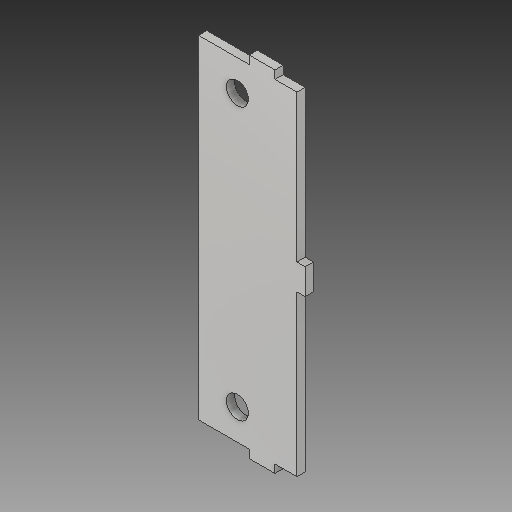
# Autodesk Inventor part: 1-8inch_Side2_2-Parts
Saved by Autodesk Inventor 2018 (Build 220112000, 112)
## iProperties
Created: 2018-02-01
Part Number: 1-8inch_Side2_2-Parts
Material: Generic
Document SubType Name: Modeling
Designer: Angie
Density: 1 g/cm^3
Appearance: Default
Author: Angie
Autodesk Inventor part; units mm, degrees
ref_plane "YZ Plane" through (0, 0, 0) normal (1, 0, 0) x (0, 1, 0)
ref_plane "XZ Plane" through (0, 0, 0) normal (0, 1, 0) x (-1, 0, 0)
ref_plane "XY Plane" through (0, 0, 0) normal (0, 0, 1) x (1, 0, 0)
sketch "Sketch1" plane through (0, 0, 0) normal (0, 0, 1) x (1, 0, 0)
  line L0 (-3, -5) -> (-3, -66.825)
  line L1 (-11.5, -67) -> (-11.5, -70)
  line L2 (-11.5, -70) -> (-21.5, -70)
  line L3 (-21.5, -70) -> (-21.5, -67)
  line L4 (-41, -66.825) -> (-41, 61.825)
  line L5 (-21.5, 61.825) -> (-21.5, 65)
  line L6 (-21.5, 65) -> (-11.5, 65)
  line L7 (-11.5, 65) -> (-11.5, 65)
  line L8 (-3, 61.825) -> (-3, 5)
  line L9 (-3, 5) -> (0, 5)
  line L10 (0, -5) -> (-3, -5)
  circle A0 centre (-26, -55) radius 4.25
  circle A1 centre (-26, 50) radius 4.25
  line L11 (-3, -5) -> (-3, -66.825)
  line L12 (-11.5, -67) -> (-11.5, -70)
  line L13 (-11.5, -70) -> (-21.5, -70)
  line L14 (-21.5, -70) -> (-21.5, -67)
  line L15 (-41, -66.825) -> (-41, 61.825)
  line L16 (-21.5, 61.825) -> (-21.5, 65)
  line L17 (-21.5, 65) -> (-11.5, 65)
  line L18 (-11.5, 65) -> (-11.5, 65)
  line L19 (-3, 61.825) -> (-3, 5)
  line L20 (-3, 5) -> (0, 5)
  line L21 (0, -5) -> (-3, -5)
  circle A2 centre (-26, -55) radius 4.25
  circle A3 centre (-26, 50) radius 4.25
  line L22 (-3, 5) -> (0.175, 5)
  line L23 (0.175, 5) -> (0.175, -5)
  line L24 (0.175, -5) -> (-3, -5)
  line L25 (-21.5, 65) -> (-11.5, 65)
  line L26 (-21.5, 65) -> (-11.5, 65)
  line L27 (-11.5, 65) -> (-11.5, 61.825)
  line L28 (-21.5, 61.825) -> (-21.5, 65)
  line L29 (-3, 61.825) -> (-11.5, 61.825)
  line L30 (-21.5, 61.825) -> (-41, 61.825)
  line L31 (-11.5, -70) -> (-11.5, -66.825)
  line L32 (-11.5, -66.825) -> (-3, -66.825)
  line L33 (-21.5, -70) -> (-21.5, -66.825)
  line L34 (-21.5, -66.825) -> (-41, -66.825)
  point P0 (0, 0)
  dimension "d0" = 3.175
  dimension "d4" = 3.175
  dimension "d5" = 3.175
  constraints: 70 end point, 5 perpendicular, 4 centre point, 4 parallel, 3 horizontal, 1 point on line
  measures "d0" distance of L23.end L0.start
  measures "d4" distance of L1.end L31.end
  measures "d5" distance of L2.end L33.end
extrude "Extrusion2" add sketch "Sketch1" along normal blind 3.175
body "Solid2"
